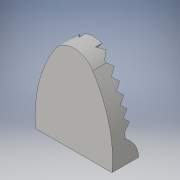
# Autodesk Inventor part: HeadFrame
Saved by Autodesk Inventor 2016 (Build 200138000, 138)
## iProperties
Created: 2017-03-13
Part Number: HeadFrame
Material: Generic
Document SubType Name: Modeling
Designer: Owner
Density: 1 g/cm^3
Appearance: Default
Author: Owner
Autodesk Inventor part; units mm, degrees
ref_plane "YZ Plane" through (0, 0, 0) normal (1, 0, 0) x (0, 1, 0)
ref_plane "XZ Plane" through (0, 0, 0) normal (0, 1, 0) x (-1, 0, 0)
ref_plane "XY Plane" through (0, 0, 0) normal (0, 0, 1) x (1, 0, 0)
sketch "Sketch1" plane through (0, 0, 0) normal (0, 0, 1) x (1, 0, 0)
  line L0 (43.1005, 62.15) -> (-43.0995, 62.15) projected
  line L1 (43.1005, 62.15) -> (-43.0995, 62.15)
  line L2 (-43.0995, 62.15) -> (-43.0995, 176.45)
  line L3 (-43.0995, 176.45) -> (43.1005, 176.45)
  line L4 (43.1005, 176.45) -> (43.1005, 62.15)
  arc A0 (43.1005, 62.15) -> (21.3887, 150.6616) centre (-96.2032, 74.8977) ccw
  arc A1 (-21.3303, 150.6382) -> (-43.0995, 62.15) centre (96.9395, 74.6204) ccw
  arc A2 (21.3887, 150.6616) -> (-21.3303, 150.6382) centre (0.0367, 136.9046) ccw
  point P0 (0, 0)
  dimension "d0" = 114.3
  dimension "d1" = 25.4
  constraints: 8 end point, 6 point on circle, 3 centre point, 2 parallel, 2 tangent, 1 horizontal, 1 perpendicular
  measures "d0" distance of L3.end L0.start
  measures "d1" radius of A2
extrude "Extrusion1" add sketch "Sketch1" against normal blind 5 contours L0 L2 A1 A2 A0 L4 | L4 A0 | A1 L2
sketch "Sketch2" plane through (0, 0, -5) normal (0, 0, -1) x (-1, 0, 0)
  arc A0 (-21.3887, 150.6616) -> (-43.1005, 62.15) centre (96.2032, 74.8977) ccw projected
  line L0 (-43.1005, 62.15) -> (43.0995, 62.15) projected
  arc A1 (43.0995, 62.15) -> (21.3303, 150.6382) centre (-96.9395, 74.6204) ccw projected
  arc A2 (21.3303, 150.6382) -> (-21.3887, 150.6616) centre (-0.0367, 136.9046) ccw projected
  arc A3 (-16.0502, 147.2223) -> (-32.7704, 90.1915) centre (72.1437, 90.3994) ccw
  arc A4 (32.7315, 90.1915) -> (15.989, 147.2048) centre (-72.7133, 90.1915) ccw
  arc A5 (15.989, 147.2048) -> (-16.0502, 147.2223) centre (-0.0363, 136.9046) ccw
  line L1 (-43.1005, 62.15) -> (43.0995, 62.15) projected
  line L2 (-32.3341, 62.15) -> (32.3159, 62.15)
  line L3 (32.7315, 90.1915) -> (32.7315, 62.15)
  line L4 (32.7315, 62.15) -> (-32.7704, 62.15)
  line L5 (-32.7704, 62.15) -> (-32.7704, 90.1915)
  point P0 (0, 0)
  constraints: 8 end point, 6 point on circle, 3 centre point, 2 point on line, 1 parallel
extrude "Extrusion2" add sketch "Sketch2" along normal blind 10 contours A2 A1 L0 L3 A4 A5 A3 L5 A0
sketch "Sketch3" plane through (-32.7315, 62.15, -5) normal (1, 0, 0) x (0, 0, -1)
  line L0 (0, 0) -> (25, 0)
  line L1 (-5, 0) -> (10, 0) projected
  line L2 (10, 0) -> (10, 25.4)
  arc A0 (25, 0) -> (10, 25.4) centre (-9.2015, -3.0686) ccw
  line L3 (10, 25.4) -> (10, -0.6619)
  line L4 (25, 0) -> (10, 0)
  line L5 (10, 0) -> (10, 25.4)
  point P0 (-5, -62.15)
  dimension "d6" = 25
  dimension "d7" = 25.4
  constraints: 10 end point, 2 collinear, 2 perpendicular, 2 point on circle, 1 centre point, 1 vertical
  measures "d6" distance of L0.start L0.end
  measures "d7" distance of L1.end L2.end
extrude "Extrusion3" add sketch "Sketch3" along normal blind 101.6 and the other way blind 25.4
sketch "Sketch4" plane through (0, 0, -15) normal (0, 0, -1) x (-1, 0, 0)
  line L0 (32.7315, 62.15) -> (32.7315, 90.1915) projected
  arc A0 (32.7315, 90.1915) -> (15.989, 147.2048) centre (-72.7133, 90.1915) ccw projected
  arc A1 (15.989, 147.2048) -> (-16.0502, 147.2223) centre (-0.0363, 136.9046) ccw projected
  arc A2 (-16.0502, 147.2223) -> (-32.7704, 90.1915) centre (72.1437, 90.3994) ccw projected
  line L1 (-32.7704, 90.1915) -> (-32.7704, 62.15) projected
  line L2 (-32.7704, 62.15) -> (32.7315, 62.15) projected
  arc A3 (-21.3887, 150.6616) -> (-43.1092, 87.55) centre (96.2032, 74.8977) ccw projected
  line L3 (-21.3887, 150.6616) -> (-130.3098, 136.9046)
  line L4 (-130.3098, 136.9046) -> (-112.8714, 20.9919)
  arc A4 (-21.3887, 150.6616) -> (-43.1005, 62.15) centre (96.2032, 74.8977) ccw projected
  line L5 (-43.1005, 62.15) -> (-112.8714, 20.9919)
  arc A5 (43.0579, 87.55) -> (21.3303, 150.6382) centre (-96.9395, 74.6204) ccw projected
  line L6 (21.3303, 150.6382) -> (115.993, 147.2223)
  line L7 (115.993, 147.2223) -> (119.9414, 13.6964)
  line L8 (119.9414, 13.6964) -> (43.0995, 62.15)
  arc A6 (43.0995, 62.15) -> (43.0579, 87.55) centre (-96.9395, 74.6204) ccw projected
  point P0 (0, 0)
  constraints: 12 end point, 1 point on circle
extrude "Extrusion4" cut sketch "Sketch4" along normal blind 25.4
sketch "Sketch5" plane through (0, 0, -15) normal (0, 0, -1) x (-1, 0, 0)
  arc A0 (15.989, 147.2048) -> (-16.0502, 147.2223) centre (-0.0363, 136.9046) ccw projected
  line L0 (32.7315, 62.15) -> (32.7315, 90.1915) projected
  arc A1 (32.7315, 90.1915) -> (15.989, 147.2048) centre (-72.7133, 90.1915) ccw projected
  arc A2 (15.989, 147.2048) -> (-16.0502, 147.2223) centre (-0.0363, 136.9046) ccw projected
  arc A3 (-16.0502, 147.2223) -> (-32.7704, 90.1915) centre (72.1437, 90.3994) ccw projected
  line L1 (-32.7704, 90.1915) -> (-32.7704, 62.15) projected
  line L2 (-32.7704, 62.15) -> (32.7315, 62.15) projected
  arc A4 (43.0579, 87.55) -> (21.3303, 150.6382) centre (-96.9395, 74.6204) ccw projected
  arc A5 (21.3303, 150.6382) -> (-21.3887, 150.6616) centre (-0.0367, 136.9046) ccw projected
  arc A6 (-21.3887, 150.6616) -> (-43.1092, 87.55) centre (96.2032, 74.8977) ccw projected
  line L3 (-0.0228, 162.3046) -> (-0.0228, 87.55)
  line L4 (-0.0228, 87.55) -> (-0.0228, 100.25)
  line L5 (-0.0228, 100.25) -> (41.2979, 100.25)
  line L6 (41.2979, 100.25) -> (-41.366, 100.25)
  line L7 (41.2979, 111.68) -> (-41.366, 111.68)
  line L8 (41.2979, 123.11) -> (-41.366, 123.11)
  line L9 (41.2979, 134.54) -> (-41.366, 134.54)
  line L10 (41.2979, 145.97) -> (-41.366, 145.97)
  line L11 (41.2979, 157.4) -> (-41.366, 157.4)
  point P0 (0, 0)
  dimension "d15" = 12.7
  dimension "d18" = 11.43
  constraints: 18 end point, 3 point on circle, 2 point on line, 2 vertical, 1 perpendicular, 15 other
  measures "d15" distance of L3.end L4.end
  measures "d18" distance of L5.end L7.start
ref_plane "Work Plane1" through (24.2822, 145.97, -15) normal (0.8613134, 0.5080741, 0) x (-0.5080741, 0.8613134, 0)
ref_plane "Work Plane2" through (30.3306, 134.54, -15) normal (0.9045515, 0.4263645, 0) x (-0.4263645, 0.9045515, 0)
ref_plane "Work Plane3" through (35.1116, 123.11, -15) normal (0.9387295, 0.3446549, 0) x (-0.3446549, 0.9387295, 0)
ref_plane "Work Plane4" through (38.76, 111.68, -15) normal (0.9648107, 0.2629453, 0) x (-0.2629453, 0.9648107, 0)
ref_plane "Work Plane5" through (41.366, 100.25, -15) normal (0.9834397, 0.1812357, 0) x (-0.1812357, 0.9834397, 0)
ref_plane "Work Plane6" through (15.04, 157.4, -15) normal (0.5906812, 0.806905, 0) x (-0.806905, 0.5906812, 0)
sketch "Sketch6" plane through (15.04, 157.4, -15) normal (0.5906812, 0.806905, 0) x (-0.806905, 0.5906812, 0)
  line L0 (0, 0) -> (-6.35, 0)
  line L1 (-9.103, 0) -> (25.4, 0) projected
  line L2 (-6.35, 0) -> (6.35, 0)
  line L3 (0, 0) -> (0, -6.35)
  line L4 (0, -6.35) -> (6.35, 0)
  line L5 (0, -6.35) -> (-6.35, 0)
  point P0 (-80.8374, 15)
  point P1 (25.3533, 0)
  dimension "d23" = 6.35
  dimension "d24" = 12.7
  dimension "d25" = 6.35
  constraints: 10 end point, 2 point on line, 1 vertical
  measures "d23" distance of L0.start L0.end
  measures "d24" distance of L0.end L2.end
  measures "d25" distance of L0.start L3.end
sketch "Sketch7" plane through (24.2822, 145.97, -15) normal (0.8613134, 0.5080741, 0) x (-0.5080741, 0.8613134, 0)
  line L0 (0, 0) -> (-6.35, 0)
  line L1 (-9.103, 0) -> (25.4, 0)
  line L2 (-6.35, 0) -> (6.35, 0)
  line L3 (0, 0) -> (0, -6.35)
  line L4 (0, -6.35) -> (6.35, 0)
  line L5 (0, -6.35) -> (-6.35, 0)
  point P0 (-113.3887, 15)
  point P1 (25.3533, 0)
  dimension "d26" = 6.35
  dimension "d27" = 12.7
  dimension "d28" = 6.35
  constraints: 12 end point, 2 point on line, 1 vertical
  measures "d26" distance of L0.start L0.end
  measures "d27" distance of L0.end L2.end
  measures "d28" distance of L0.start L3.end
sketch "Sketch8" plane through (30.3306, 134.54, -15) normal (0.9045515, 0.4263645, 0) x (-0.4263645, 0.9045515, 0)
  line L0 (0, 0) -> (-6.35, 0)
  line L1 (-9.103, 0) -> (25.4, 0)
  line L2 (-6.35, 0) -> (6.35, 0)
  line L3 (0, 0) -> (0, -6.35)
  line L4 (0, -6.35) -> (6.35, 0)
  line L5 (0, -6.35) -> (-6.35, 0)
  point P0 (-108.7665, 15)
  point P1 (25.3533, 0)
  dimension "d29" = 6.35
  dimension "d30" = 12.7
  dimension "d31" = 6.35
  constraints: 12 end point, 2 point on line, 1 vertical
  measures "d29" distance of L0.start L0.end
  measures "d30" distance of L0.end L2.end
  measures "d31" distance of L0.start L3.end
sketch "Sketch9" plane through (35.1116, 123.11, -15) normal (0.9387295, 0.3446549, 0) x (-0.3446549, 0.9387295, 0)
  line L0 (0, 0) -> (-6.35, 0)
  line L1 (-9.103, 0) -> (25.4, 0)
  line L2 (-6.35, 0) -> (6.35, 0)
  line L3 (0, 0) -> (0, -6.35)
  line L4 (0, -6.35) -> (6.35, 0)
  line L5 (0, -6.35) -> (-6.35, 0)
  point P0 (-103.4656, 15)
  point P1 (25.3533, 0)
  dimension "d32" = 6.35
  dimension "d33" = 12.7
  dimension "d34" = 6.35
  constraints: 12 end point, 2 point on line, 1 vertical
  measures "d32" distance of L0.start L0.end
  measures "d33" distance of L0.end L2.end
  measures "d34" distance of L0.start L3.end
sketch "Sketch10" plane through (38.76, 111.68, -15) normal (0.9648107, 0.2629453, 0) x (-0.2629453, 0.9648107, 0)
  line L0 (0, 0) -> (-6.35, 0)
  line L1 (-9.103, 0) -> (25.4, 0)
  line L2 (-6.35, 0) -> (6.35, 0)
  line L3 (0, 0) -> (0, -6.35)
  line L4 (0, -6.35) -> (6.35, 0)
  line L5 (0, -6.35) -> (-6.35, 0)
  point P0 (-97.5583, 15)
  point P1 (25.3533, 0)
  dimension "d35" = 6.35
  dimension "d36" = 12.7
  dimension "d37" = 6.35
  constraints: 12 end point, 2 point on line, 1 vertical
  measures "d35" distance of L0.start L0.end
  measures "d36" distance of L0.end L2.end
  measures "d37" distance of L0.start L3.end
sketch "Sketch11" plane through (41.366, 100.25, -15) normal (0.9834397, 0.1812357, 0) x (-0.1812357, 0.9834397, 0)
  line L0 (0, 0) -> (-6.35, 0)
  line L1 (-9.103, 0) -> (25.4, 0)
  line L2 (-6.35, 0) -> (6.35, 0)
  line L3 (0, 0) -> (0, -6.35)
  line L4 (0, -6.35) -> (6.35, 0)
  line L5 (0, -6.35) -> (-6.35, 0)
  point P0 (-91.0928, 15)
  point P1 (25.3533, 0)
  dimension "d38" = 6.35
  dimension "d39" = 12.7
  dimension "d40" = 6.35
  constraints: 12 end point, 2 point on line, 1 vertical
  measures "d38" distance of L0.start L0.end
  measures "d39" distance of L0.end L2.end
  measures "d40" distance of L0.start L3.end
extrude "Extrusion5" add sketch "Sketch7" against normal blind 25.4
extrude "Extrusion6" add sketch "Sketch6" against normal blind 25.4
extrude "Extrusion7" add sketch "Sketch8" against normal blind 25.4
extrude "Extrusion8" add sketch "Sketch9" against normal blind 25.4
extrude "Extrusion9" add sketch "Sketch10" against normal blind 25.4
extrude "Extrusion10" add sketch "Sketch11" against normal blind 25.4
ref_plane "Work Plane7" through (-14.9666, 157.4, -15) normal (-0.5906812, 0.806905, 0) x (-0.806905, -0.5906812, 0)
ref_plane "Work Plane8" through (-24.2037, 145.97, -15) normal (-0.8616578, 0.5074897, 0) x (-0.5074897, -0.8616578, 0)
ref_plane "Work Plane9" through (-30.2458, 134.54, -15) normal (-0.9046331, 0.4261913, 0) x (-0.4261913, -0.9046331, 0)
ref_plane "Work Plane10" through (-35.0272, 123.11, -15) normal (-0.938642, 0.3448929, 0) x (-0.3448929, -0.938642, 0)
ref_plane "Work Plane11" through (-38.6814, 111.68, -15) normal (-0.9646336, 0.2635945, 0) x (-0.2635945, -0.9646336, 0)
ref_plane "Work Plane12" through (-41.2979, 100.25, -15) normal (-0.9832437, 0.1822961, 0) x (-0.1822961, -0.9832437, 0)
sketch "Sketch13" plane through (-14.9666, 157.4, -15) normal (-0.5906812, 0.806905, 0) x (-0.806905, -0.5906812, 0)
  line L0 (0, 0) -> (-6.35, 0)
  line L1 (6.8471, 0) -> (-15.2018, 0) projected
  line L2 (-6.35, 0) -> (6.35, 0)
  line L3 (0, 0) -> (0, -6.35)
  line L4 (0, -6.35) -> (-6.35, 0)
  line L5 (0, -6.35) -> (6.35, 0)
  point P0 (80.8966, 15)
  dimension "d56" = 6.35
  dimension "d57" = 12.7
  dimension "d58" = 6.35
  constraints: 10 end point, 2 point on line, 1 vertical
  measures "d56" distance of L0.start L0.end
  measures "d57" distance of L0.end L2.end
  measures "d58" distance of L0.start L3.end
sketch "Sketch14" plane through (-24.2037, 145.97, -15) normal (-0.8616578, 0.5074897, 0) x (-0.5074897, -0.8616578, 0)
  line L0 (0, 0) -> (-6.35, 0)
  line L1 (6.8467, 0) -> (-15.2019, 0)
  line L2 (-6.35, 0) -> (6.35, 0)
  line L3 (0, 0) -> (0, -6.35)
  line L4 (0, -6.35) -> (-6.35, 0)
  line L5 (0, -6.35) -> (6.35, 0)
  point P0 (113.493, 15)
  dimension "d59" = 6.35
  dimension "d60" = 12.7
  dimension "d61" = 6.35
  constraints: 12 end point, 2 point on line, 1 vertical
  measures "d59" distance of L0.start L0.end
  measures "d60" distance of L0.end L2.end
  measures "d61" distance of L0.start L3.end
sketch "Sketch15" plane through (-30.2458, 134.54, -15) normal (-0.9046331, 0.4261913, 0) x (-0.4261913, -0.9046331, 0)
  line L0 (0, 0) -> (-6.35, 0)
  line L1 (6.8467, 0) -> (-15.2019, 0)
  line L2 (-6.35, 0) -> (6.35, 0)
  line L3 (0, 0) -> (0, -6.35)
  line L4 (0, -6.35) -> (-6.35, 0)
  line L5 (0, -6.35) -> (6.35, 0)
  point P0 (108.8189, 15)
  dimension "d62" = 6.35
  dimension "d63" = 12.7
  dimension "d64" = 6.35
  constraints: 12 end point, 2 point on line, 1 vertical
  measures "d62" distance of L0.start L0.end
  measures "d63" distance of L0.end L2.end
  measures "d64" distance of L0.start L3.end
sketch "Sketch16" plane through (-35.0272, 123.11, -15) normal (-0.938642, 0.3448929, 0) x (-0.3448929, -0.938642, 0)
  line L0 (0, 0) -> (-6.35, 0)
  line L1 (6.8467, 0) -> (-15.2019, 0)
  line L2 (-6.35, 0) -> (6.35, 0)
  line L3 (0, 0) -> (0, -6.35)
  line L4 (0, -6.35) -> (-6.35, 0)
  line L5 (0, -6.35) -> (6.35, 0)
  point P0 (103.4756, 15)
  dimension "d65" = 6.35
  dimension "d66" = 12.7
  dimension "d67" = 6.35
  constraints: 12 end point, 2 point on line, 1 vertical
  measures "d65" distance of L0.start L0.end
  measures "d66" distance of L0.end L2.end
  measures "d67" distance of L0.start L3.end
sketch "Sketch17" plane through (-38.6814, 111.68, -15) normal (-0.9646336, 0.2635945, 0) x (-0.2635945, -0.9646336, 0)
  line L0 (0, 0) -> (-6.35, 0)
  line L1 (6.8467, 0) -> (-15.2019, 0)
  line L2 (-6.35, 0) -> (6.35, 0)
  line L3 (0, 0) -> (0, -6.35)
  line L4 (0, -6.35) -> (-6.35, 0)
  line L5 (0, -6.35) -> (6.35, 0)
  point P0 (97.5341, 15)
  dimension "d68" = 6.35
  dimension "d69" = 12.7
  dimension "d70" = 6.35
  constraints: 12 end point, 2 point on line, 1 vertical
  measures "d68" distance of L0.start L0.end
  measures "d69" distance of L0.end L2.end
  measures "d70" distance of L0.start L3.end
sketch "Sketch18" plane through (-41.2979, 100.25, -15) normal (-0.9832437, 0.1822961, 0) x (-0.1822961, -0.9832437, 0)
  line L0 (0, 0) -> (-6.35, 0)
  line L1 (6.8467, 0) -> (-15.2019, 0)
  line L2 (-6.35, 0) -> (6.35, 0)
  line L3 (0, 0) -> (0, -6.35)
  line L4 (0, -6.35) -> (-6.35, 0)
  line L5 (0, -6.35) -> (6.35, 0)
  point P0 (91.0417, 15)
  dimension "d71" = 6.35
  dimension "d72" = 12.7
  dimension "d73" = 6.35
  constraints: 12 end point, 2 point on line, 1 vertical
  measures "d71" distance of L0.start L0.end
  measures "d72" distance of L0.end L2.end
  measures "d73" distance of L0.start L3.end
extrude "Extrusion11" add sketch "Sketch13" against normal blind 25.4
extrude "Extrusion12" add sketch "Sketch14" against normal blind 25.4
extrude "Extrusion13" add sketch "Sketch15" against normal blind 25.4
extrude "Extrusion14" add sketch "Sketch16" against normal blind 25.4
extrude "Extrusion15" add sketch "Sketch17" against normal blind 25.4
extrude "Extrusion16" add sketch "Sketch18" against normal blind 25.4
sketch "Sketch19" plane through (0, 0, -5) normal (0, 0, -1) x (-1, 0, 0)
  line L0 (32.7315, 62.15) -> (32.7315, 90.1915) projected
  arc A0 (32.7315, 90.1915) -> (15.989, 147.2048) centre (-72.7133, 90.1915) ccw projected
  arc A1 (15.989, 147.2048) -> (-16.0502, 147.2223) centre (-0.0363, 136.9046) ccw projected
  arc A2 (-16.0502, 147.2223) -> (-32.7704, 90.1915) centre (72.1437, 90.3994) ccw projected
  line L1 (-32.7704, 90.1915) -> (-32.7704, 62.15) projected
  line L2 (-32.7704, 62.15) -> (32.7315, 62.15) projected
  point P0 (0, 0)
extrude "Extrusion17" cut sketch "Sketch19" along normal blind 25.4
sketch "Sketch20" plane through (0, 0, 0) normal (0, 0, 1) x (1, 0, 0)
  arc A0 (21.3887, 150.6616) -> (-21.3303, 150.6382) centre (0.0367, 136.9046) ccw projected
  arc A1 (-21.3303, 150.6382) -> (-43.0995, 62.15) centre (96.9395, 74.6204) ccw projected
  arc A2 (43.1005, 62.15) -> (21.3887, 150.6616) centre (-96.2032, 74.8977) ccw projected
  line L0 (43.1005, 62.15) -> (-43.0995, 62.15) projected
  line L1 (-43.0995, 62.15) -> (-82.9194, 62.15)
  line L2 (-82.9194, 62.15) -> (-48.8807, 239.8541)
  line L3 (-48.8807, 239.8541) -> (69.4632, 239.8541)
  line L4 (69.4632, 239.8541) -> (43.1005, 62.15)
  point P0 (0, 0)
  constraints: 8 end point, 1 horizontal, 1 parallel
extrude "Extrusion18" cut sketch "Sketch20" against normal blind 101.6 contours A0 A1 L1 L2 L3 L4 A2
sketch "Sketch21" plane through (0, 0, -5) normal (0, 0, -1) x (-1, 0, 0)
  line L0 (4.8495, 69.64) -> (-4.8505, 69.64) projected
  line L1 (-4.8505, 68.6) -> (4.8495, 68.6) projected
  line L2 (4.8495, 69.64) -> (4.8495, 79.64)
  line L3 (-4.8505, 69.64) -> (-4.8505, 79.64)
  line L4 (4.8495, 79.64) -> (6.8495, 79.64)
  line L5 (-4.8505, 79.64) -> (-6.8505, 79.64)
  line L6 (6.8495, 79.64) -> (11.8495, 79.64)
  line L7 (11.8495, 79.64) -> (11.8495, 99.64)
  line L8 (11.8495, 99.64) -> (6.8495, 99.64)
  line L9 (6.8495, 99.64) -> (6.8495, 79.64)
  line L10 (-6.8505, 79.64) -> (-11.8505, 79.64)
  line L11 (-11.8505, 79.64) -> (-11.8505, 99.64)
  line L12 (-11.8505, 99.64) -> (-6.8505, 99.64)
  line L13 (-6.8505, 99.64) -> (-6.8505, 79.64)
  point P0 (0, 0)
  dimension "d90" = 10
  dimension "d91" = 10
  dimension "d92" = 2
  dimension "d93" = 2
  dimension "d94" = 5
  dimension "d95" = 20
  dimension "d96" = 5
  dimension "d97" = 20
  constraints: 24 end point, 4 horizontal, 4 parallel, 2 perpendicular, 2 vertical
  measures "d90" distance of L0.start L2.end
  measures "d91" distance of L0.end L3.end
  measures "d92" distance of L2.end L4.end
  measures "d93" distance of L3.end L5.end
  measures "d94" distance of L7.end L8.end
  measures "d95" distance of L6.end L7.end
  measures "d96" distance of L11.end L12.end
  measures "d97" distance of L10.end L11.end
extrude "Extrusion19" add sketch "Sketch21" along normal blind 31.5
sketch "Sketch22" plane through (-11.8495, 79.64, -5) normal (-1, 0, 0) x (0, 0, 1)
  line L0 (-31.5, 0) -> (-31.5, 20) projected
  line L1 (-31.5, 10) -> (-26.5, 10)
  circle A0 centre (-26.5, 10) radius 1.75
  point P0 (5, -79.64)
  dimension "d100" = 5
  dimension "d101" = 3.5
  constraints: 2 end point, 1 centre point, 1 coincident, 1 horizontal, 1 midpoint
  measures "d100" distance of L1.start L1.end
  measures "d101" diameter of A0
extrude "Extrusion20" cut sketch "Sketch22" against normal blind 40
sketch "Sketch23" plane through (0, 0, -5) normal (0, 0, -1) x (-1, 0, 0)
  line L0 (-6.8505, 79.64) -> (-11.8505, 79.64) projected
  line L1 (-11.8505, 79.64) -> (-11.8505, 99.64) projected
  line L2 (-11.8505, 99.64) -> (-6.8505, 99.64) projected
  line L3 (-6.8505, 99.64) -> (-6.8505, 79.64) projected
  line L4 (6.8495, 79.64) -> (6.8495, 99.64) projected
  line L5 (6.8495, 99.64) -> (11.8495, 99.64) projected
  line L6 (11.8495, 99.64) -> (11.8495, 79.64) projected
  line L7 (11.8495, 79.64) -> (6.8495, 79.64) projected
  line L8 (32.7315, 62.15) -> (32.7315, 90.1915) projected
  arc A0 (32.7315, 90.1915) -> (15.989, 147.2048) centre (-72.7133, 90.1915) ccw projected
  arc A1 (15.989, 147.2048) -> (-16.0502, 147.2223) centre (-0.0363, 136.9046) ccw projected
  arc A2 (-16.0502, 147.2223) -> (-32.7704, 90.1915) centre (72.1437, 90.3994) ccw projected
  line L9 (-32.7704, 90.1915) -> (-32.7704, 62.15) projected
  line L10 (-32.7704, 62.15) -> (32.7315, 62.15) projected
  line L11 (37.6467, 50.9368) -> (37.6467, 83.1845)
  arc A3 (37.6467, 83.1845) -> (18.3928, 148.7499) centre (-83.6149, 83.1845) ccw
  arc A4 (18.3928, 148.7499) -> (-18.4523, 148.77) centre (-0.0363, 136.9046) ccw
  arc A5 (-18.4523, 148.77) -> (-37.6805, 83.1845) centre (82.9706, 83.4237) ccw
  line L12 (-37.6805, 83.1845) -> (-37.6805, 50.9368)
  line L13 (-37.6805, 50.9368) -> (37.6467, 50.9368)
  line L14 (-6.8505, 79.64) -> (-6.8505, 99.64) projected
  line L15 (-6.8505, 99.64) -> (-11.8505, 99.64) projected
  line L16 (-11.8505, 99.64) -> (-11.8505, 79.64) projected
  line L17 (-11.8505, 79.64) -> (-6.8505, 79.64) projected
  line L18 (6.8495, 79.64) -> (11.8495, 79.64) projected
  line L19 (11.8495, 79.64) -> (11.8495, 99.64) projected
  line L20 (11.8495, 99.64) -> (6.8495, 99.64) projected
  line L21 (6.8495, 99.64) -> (6.8495, 79.64) projected
  point P0 (0, 0)
  constraints: 6 end point, 6 point on circle, 3 centre point
extrude "Extrusion21" cut sketch "Sketch23" along normal blind 40 contours L13 L12 A5 A4 A3 L11
sketch "Sketch24" plane through (0, 0, -15) normal (0, 0, -1) x (-1, 0, 0)
  arc A0 (7.2244, 157.574) -> (-7.2976, 157.5737) centre (-0.0363, 136.9046) ccw projected
  line L0 (7.2244, 157.574) -> (9.3663, 160.5) projected
  arc A1 (9.3663, 160.5) -> (-9.4398, 160.5) centre (-0.0367, 136.9046) ccw projected
  line L1 (-9.4398, 160.5) -> (-7.2976, 157.5737) projected
  point P0 (0, 0)
extrude "Extrusion22" add sketch "Sketch24" along normal blind 7.5
body "Solid1"
